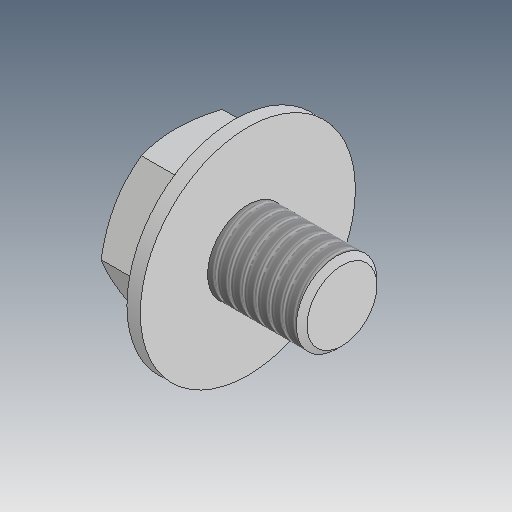
# Autodesk Inventor part: Bolt3W
Saved by Autodesk Inventor 2017 (Build 210142000, 142)
## iProperties
Created: 2010-08-06
Part Number: Bolt3W
Document SubType Name: Modeling
Designer: nguyenducthang
Density: 1 g/cm^3
Mass: 0.101983 g
Surface Area: 1.83556 cm^2
Volume: 0.101983 cm^3
Material: Generic
Appearance: Default
Author: nguyenducthang
Autodesk Inventor part; units mm, degrees
ref_plane "YZ Plane" through (0, 0, 0) normal (1, 0, 0) x (0, 1, 0)
ref_plane "XZ Plane" through (0, 0, 0) normal (0, 1, 0) x (-1, 0, 0)
ref_plane "XY Plane" through (0, 0, 0) normal (0, 0, 1) x (1, 0, 0)
sketch "Sketch15" plane through (0, 0, 0) normal (0, 0, 1) x (1, 0, 0)
  line L0 (0, 0) -> (0, 2.5)
  line L1 (0.2887, 3) -> (2.25, 3)
  line L2 (3, 4.4) -> (3, 4.4)
  line L3 (2.25, 1.5) -> (6.25, 1.5)
  line L4 (6.25, 0) -> (0, 0)
  line L5 (0.2887, 3) -> (0, 2.5)
  line L6 (2.25, 1.5) -> (2.25, 3)
  line L7 (6.25, 1.5) -> (6.25, 0)
  dimension "d83" = 30
  dimension "d84" = 1.5
  dimension "d86" = 0.5
  dimension "d87" = 3
  dimension "d116" = 2.25
  dimension "d117" = 4
  constraints: 16 end point, 4 parallel, 1 perpendicular, 1 vertical, 1 other
  measures "d83" angle of L0 L5
  measures "d84" distance between parallel lines of L3 L4
  measures "d86" distance from line of L0.end L1
  measures "d87" distance between parallel lines of L1 L4
  measures "d116" distance between parallel lines of L0 L6
  measures "d117" distance of L3.start L3.end
revolve "Revolution1" add sketch "Sketch15" angle 360 about axis through (6.25, 0, 0) along (-1, 0, 0)
sketch "Sketch16" plane through (0, 0, 0) normal (-1, 0, 0) x (0, 0, 1)
  circle A0 centre (0, 0) radius 2.5 projected
  line L0 (1.5, 2.5981) -> (3, 0)
  line L1 (3, 0) -> (1.5, -2.5981)
  line L2 (1.5, -2.5981) -> (-1.5, -2.5981)
  line L3 (-1.5, -2.5981) -> (-3, 0)
  line L4 (-3, 0) -> (-1.5, 2.5981)
  line L5 (-1.5, 2.5981) -> (1.5, 2.5981)
  circle A1 centre (0, 0) radius 5.2707
  dimension "d128" = 3
  constraints: 12 end point, 2 coincident, 1 centre point, 13 other
  measures "d128" distance of L4.end L0.start
extrude "Extrusion15" cut sketch "Sketch16" against normal blind 5 contours A1
chamfer "Chamfer5" distance 0.2 angle 45 1 edges at (6.25, -1.5, 0)
thread "Thread7" size "M3x0.5" class "6g" standard "ANSI Metric M Profile" full length
sketch "Sketch19" plane through (2.25, -2.5981, 1.5) normal (1, 0, 0) x (0, 0, -1)
  circle A0 centre (1.5, 2.5981) radius 1.5 projected
  circle A1 centre (1.5, 2.5981) radius 4
  dimension "d131" = 8
  constraints: 1 centre point
  measures "d131" diameter of A1
extrude "Extrusion18" add sketch "Sketch19" along normal blind 0.5
body "Solid1"
